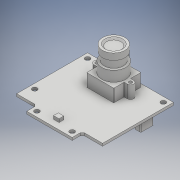
# Autodesk Inventor part: PixyCMUcam5
Saved by Autodesk Inventor 2018 (Build 220112000, 112)
## iProperties
Created: 2017-11-10
Part Number: PixyCMUcam5
Material: Generic
Document SubType Name: Modeling
Designer: leo2a
Density: 1 g/cm^3
Appearance: Default
Author: leo2a
Autodesk Inventor part; units mm, degrees
ref_plane "YZ Plane" through (0, 0, 0) normal (1, 0, 0) x (0, 1, 0)
ref_plane "XZ Plane" through (0, 0, 0) normal (0, 1, 0) x (-1, 0, 0)
ref_plane "XY Plane" through (0, 0, 0) normal (0, 0, 1) x (1, 0, 0)
sketch "Sketch1" plane through (0, 0, 0) normal (0, 0, 1) x (1, 0, 0)
  line L0 (-26.924, 25.4) -> (26.924, 25.4)
  line L1 (-26.924, 25.4) -> (-26.924, -19.05)
  line L2 (-14.224, -25.4) -> (-14.224, -20.32)
  line L3 (-15.494, -19.05) -> (-26.924, -19.05)
  line L4 (26.924, 25.4) -> (26.924, -19.05)
  line L5 (26.924, -19.05) -> (15.494, -19.05)
  line L6 (14.224, -20.32) -> (14.224, -25.4)
  line L7 (14.224, -25.4) -> (-14.224, -25.4)
  line L8 (-15.494, -19.05) -> (-14.224, -20.32)
  line L9 (14.224, -20.32) -> (15.494, -19.05)
  point P0 (0, 0)
  point P1 (-14.224, -19.05)
  point P2 (14.224, -19.05)
  dimension "d7" = 1.27
  dimension "d8" = 1.27
  dimension "d9" = 1.27
  dimension "d10" = 1.27
  constraints: 20 end point, 4 perpendicular, 4 point on line, 2 vertical
  measures "d7" distance of L3.start point (-14.224, -19.05)
  measures "d8" distance of L2.end point (-14.224, -19.05)
  measures "d9" distance of L6.start point (14.224, -19.05)
  measures "d10" distance of L5.end point (14.224, -19.05)
extrude "Extrusion1" add sketch "Sketch1" along normal blind 1.6
sketch "Sketch2" plane through (0, 0, 1.6) normal (0, 0, 1) x (1, 0, 0)
  line L0 (26.924, 25.4) -> (-26.924, 25.4) projected
  line L1 (-26.924, 25.4) -> (-26.924, 22.225)
  line L2 (-26.924, 25.4) -> (-26.924, -19.05) projected
  line L3 (-26.924, 22.225) -> (-23.749, 22.225)
  line L4 (26.924, 22.225) -> (23.749, 22.225)
  line L5 (14.224, -25.4) -> (-14.224, -25.4) projected
  line L6 (-14.224, -25.4) -> (-11.049, -25.4)
  line L7 (-11.049, -25.4) -> (-11.049, -22.225)
  line L8 (14.224, -25.4) -> (11.049, -25.4)
  line L9 (11.049, -25.4) -> (11.049, -22.225)
  line L10 (-26.924, -19.05) -> (-26.924, -10.922)
  line L11 (-26.924, -10.922) -> (-23.749, -10.922)
  point P0 (0, 0)
  dimension "d13" = 3.175
  dimension "d14" = 3.175
  dimension "d15" = 3.175
  dimension "d16" = 3.175
  dimension "d17" = 3.175
  dimension "d18" = 3.175
  dimension "d19" = 8.128
  dimension "d20" = 3.175
  constraints: 18 end point, 6 coincident, 4 perpendicular, 4 point on line, 1 horizontal
  measures "d13" distance of L0.end L1.end
  measures "d14" distance of L1.end L3.end
  measures "d15" distance of L4.start L4.end
  measures "d16" distance of L5.end L6.end
  measures "d17" distance of L6.end L7.end
  measures "d18" distance of L5.start L8.end
  measures "d19" distance of L2.end L10.end
  measures "d20" distance of L10.end L11.end
hole "Hole1" at (-23.749, 22.225, 1.6) at (23.749, 22.225, 1.6) at (-11.049, -22.225, 1.6) at (11.049, -22.225, 1.6) at (-23.749, -10.922, 1.6) direction (0, 0, -1) diameter 3.048 end through all
sketch "Sketch3" plane through (0, 0, 1.6) normal (0, 0, 1) x (1, 0, 0)
  line L0 (-26.924, 25.4) -> (26.924, 25.4) projected
  line L1 (0, 23.4) -> (8.5, 23.4)
  line L2 (8.5, 23.4) -> (8.5, 16.9)
  line L3 (8.5, 6.4) -> (-8.5, 6.4)
  line L4 (-8.5, 6.4) -> (-8.5, 12.9)
  line L5 (-8.5, 23.4) -> (0, 23.4)
  line L6 (-8.5, 23.4) -> (-8.5, 16.9)
  line L7 (-8.5, 12.9) -> (-10.5, 12.9)
  line L8 (-12.5, 14.9) -> (-12.5, 14.9)
  line L9 (-10.5, 16.9) -> (-8.5, 16.9)
  line L10 (-8.5, 16.9) -> (-8.5, 23.4)
  line L11 (8.5, 12.9) -> (10.5, 12.9)
  line L12 (12.5, 14.9) -> (12.5, 14.9)
  line L13 (10.5, 16.9) -> (8.5, 16.9)
  line L14 (8.5, 12.9) -> (8.5, 6.4)
  arc A0 (-10.5, 16.9) -> (-12.5, 14.9) centre (-10.5, 14.9) ccw
  arc A1 (-12.5, 14.9) -> (-10.5, 12.9) centre (-10.5, 14.9) ccw
  arc A2 (10.5, 12.9) -> (12.5, 14.9) centre (10.5, 14.9) ccw
  arc A3 (12.5, 14.9) -> (10.5, 16.9) centre (10.5, 14.9) ccw
  point P0 (0, 0)
  dimension "d35" = 2
  constraints: 28 end point, 9 perpendicular, 8 point on circle, 8 tangent, 4 centre point, 3 equal radius, 1 collinear, 1 horizontal, 1 point on line
  measures "d35" radius of A0
extrude "Extrusion2" add sketch "Sketch3" along normal blind 8
sketch "Sketch4" plane through (0, 0, 9.6) normal (0, 0, 1) x (1, 0, 0)
  circle A0 centre (0, 14.9) radius 7.5
  point P0 (0, 0)
  dimension "d38" = 15
  constraints: 1 centre point
  measures "d38" diameter of A0
extrude "Extrusion3" add sketch "Sketch4" along normal blind 6.5
sketch "Sketch5" plane through (0, 14.9, 16.1) normal (0, 0, 1) x (1, 0, 0)
  circle A0 centre (0, 0) radius 6
  point P0 (0, -14.9)
  dimension "d41" = 12
  constraints: 1 centre point
  measures "d41" diameter of A0
extrude "Extrusion4" add sketch "Sketch5" along normal blind 5
sketch "Sketch6" plane through (0, 14.9, 21.1) normal (0, 0, 1) x (1, 0, 0)
  circle A0 centre (0, 0) radius 7
  point P0 (0, -14.9)
  dimension "d44" = 14
  constraints: 1 centre point
  measures "d44" diameter of A0
extrude "Extrusion5" add sketch "Sketch6" along normal blind 4
sketch "Sketch7" plane through (0, 14.9, 25.1) normal (0, 0, 1) x (1, 0, 0)
  circle A0 centre (0, 0) radius 5.5
  point P0 (0, -14.9)
  dimension "d47" = 11
  constraints: 1 centre point
  measures "d47" diameter of A0
extrude "Extrusion6" cut sketch "Sketch7" against normal blind 1
chamfer "Chamfer1" distance 1 angle 45 1 edges at (-5.5, 14.9, 24.1)
sketch "Sketch8" plane through (0, 0, 9.6) normal (0, 0, 1) x (1, 0, 0)
  line L0 (-8.5, 23.4) -> (8.5, 23.4) projected
  line L1 (0, 23.4) -> (1.25, 23.4)
  line L2 (1.25, 23.4) -> (1.25, 22.2951)
  line L3 (0, 23.4) -> (-1.25, 23.4)
  line L4 (-1.25, 23.4) -> (-1.25, 22.2951)
  arc A0 (-1.25, 22.2951) -> (1.25, 22.2951) centre (0, 14.9) ccw
  arc A1 (1.25, 22.2951) -> (-1.25, 22.2951) centre (0, 14.9) ccw
  point P0 (0, 0)
  dimension "d53" = 1.25
  dimension "d54" = 1.25
  constraints: 8 end point, 4 point on circle, 2 centre point, 2 perpendicular, 2 point on line, 1 coincident, 1 midpoint
  measures "d53" distance of L1.start L1.end
  measures "d54" distance of L1.start L3.end
extrude "Extrusion7" add sketch "Sketch8" along normal up to surface (6.5 mm away) contours L0 L2 A1 L4
sketch "Sketch9" plane through (-8.5, 23.4, 1.6) normal (0, 1, 0) x (1, 0, 0)
  line L0 (7.25, -14.5) -> (9.75, -14.5) projected
  line L1 (8.5, -14.5) -> (8.5, -11.5)
  point P0 (8.5, 1.6)
  dimension "d57" = 3
  constraints: 2 end point, 1 coincident, 1 midpoint, 1 vertical
  measures "d57" distance of L1.start L1.end
hole "Hole2" at (0, 23.4, 13.1) direction (0, -1, 0) diameter 1.25 depth 3
sketch "Sketch10" plane through (0, 0, 9.6) normal (0, 0, 1) x (1, 0, 0)
  arc A0 (-10.5, 16.9) -> (-10.5, 12.9) centre (-10.5, 14.9) ccw projected
  arc A1 (10.5, 12.9) -> (10.5, 16.9) centre (10.5, 14.9) ccw projected
  point P0 (0, 0)
  constraints: 2 coincident
hole "Hole3" at (-10.5, 14.9, 9.6) at (10.5, 14.9, 9.6) direction (0, 0, -1) diameter 2 depth 8
sketch "Sketch11" plane through (0, 0, 0) normal (0, 0, -1) x (-1, 0, 0)
  line L0 (26.924, 25.4) -> (26.924, -19.05) projected
  line L1 (26.924, 25.4) -> (26.924, 24.4)
  line L2 (26.924, 24.4) -> (21.924, 24.4)
  line L3 (21.924, 24.4) -> (21.924, 4.4)
  line L4 (21.924, 4.4) -> (12.924, 4.4)
  line L5 (12.924, 4.4) -> (12.924, 24.4)
  line L6 (12.924, 24.4) -> (21.924, 24.4)
  point P0 (0, 0)
  dimension "d72" = 1
  dimension "d73" = 5
  dimension "d74" = 20
  dimension "d75" = 9
  constraints: 12 end point, 5 perpendicular, 2 point on line
  measures "d72" distance of L0.start L1.end
  measures "d73" distance of L1.end L2.end
  measures "d74" distance of L2.end L3.end
  measures "d75" distance of L3.end L4.end
extrude "Extrusion8" add sketch "Sketch11" along normal blind 10
sketch "Sketch13" plane through (0, 0, 0) normal (0, 0, -1) x (-1, 0, 0)
  line L0 (-26.924, 25.4) -> (26.924, 25.4) projected
  line L1 (-26.924, 25.4) -> (-21.924, 25.4)
  line L2 (-21.924, 25.4) -> (-21.924, 17.9)
  line L3 (-21.924, 17.9) -> (-17.924, 17.9)
  line L4 (-17.924, 17.9) -> (-17.924, 9.9)
  line L5 (-17.924, 9.9) -> (-21.924, 9.9)
  line L6 (-21.924, 9.9) -> (-21.924, 17.9)
  point P0 (0, 0)
  dimension "d78" = 5
  dimension "d79" = 7.5
  dimension "d80" = 4
  dimension "d81" = 8
  constraints: 12 end point, 2 parallel, 2 perpendicular, 1 horizontal, 1 point on line
  measures "d78" distance of L0.start L1.end
  measures "d79" distance of L1.end L2.end
  measures "d80" distance of L2.end L3.end
  measures "d81" distance of L3.end L4.end
extrude "Extrusion9" add sketch "Sketch13" along normal blind 9.5
fillet "Fillet1" radius 0.5 4 edges at (21.924, 17.9, -4.75) (21.924, 9.9, -4.75) (17.924, 9.9, -4.75) (17.924, 17.9, -4.75)
sketch "Sketch14" plane through (0, 0, 1.6) normal (0, 0, 1) x (1, 0, 0)
  line L0 (-14.224, -25.4) -> (-14.224, -20.32) projected
  line L1 (-14.224, -25.4) -> (-1.524, -25.4)
  line L2 (14.224, -25.4) -> (-14.224, -25.4) projected
  line L3 (-1.524, -25.4) -> (-1.524, -21.4)
  line L4 (-1.524, -21.4) -> (1.976, -21.4)
  line L5 (1.976, -21.4) -> (1.976, -18.4)
  line L6 (1.976, -18.4) -> (-1.524, -18.4)
  line L7 (-1.524, -18.4) -> (-1.524, -21.4)
  point P0 (0, 0)
  dimension "d85" = 12.7
  dimension "d86" = 4
  dimension "d87" = 3.5
  dimension "d88" = 3
  constraints: 12 end point, 2 parallel, 1 horizontal, 1 perpendicular, 1 point on line, 1 vertical
  measures "d85" distance of L0.start L1.end
  measures "d86" distance of L1.end L3.end
  measures "d87" distance of L3.end L4.end
  measures "d88" distance of L5.end L4.end
extrude "Extrusion10" add sketch "Sketch14" along normal blind 2
fillet "Fillet2" radius 0.25 10 edges at (1.25, 22.2951, 12.85) (-1.25, 22.2951, 12.85) (8.5, 23.4, 5.6) (8.5, 16.9, 5.6) (8.5, 6.4, 5.6) (-8.5, 23.4, 5.6) (-8.5, 16.9, 5.6) (-8.5, 12.9, 5.6) (8.5, 12.9, 5.6) (-8.5, 6.4, 5.6)
equation "\"d8\" = d7"
equation "\"d9\" = d7"
equation "\"d10\" = d9"
body "Solid1"
